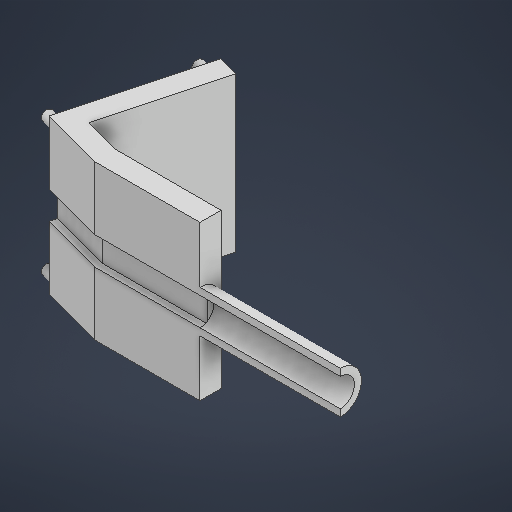
# Autodesk Inventor part: GY_906 Casetop
Saved by Autodesk Inventor 2027.1 (Build 311270010, 270A)
## iProperties
Created: 2026-09-10
Part Number: GY_906 Casetop
Material: Genérico
Document SubType Name: Modeling
Designer: marco
Density: 1 g/cm^3
Appearance: Valor por defecto
Author: marco
Autodesk Inventor part; units mm, degrees
ref_plane "YZ Plane" through (0, 0, 0) normal (1, 0, 0) x (0, 1, 0)
ref_plane "XZ Plane" through (0, 0, 0) normal (0, 1, 0) x (-1, 0, 0)
ref_plane "XY Plane" through (0, 0, 0) normal (0, 0, 1) x (1, 0, 0)
sketch "Boceto1" plane through (0, 0, 0) normal (0, 1, 0) x (-1, 0, 0)
  line L0 (0, 0) -> (-15, 0)
  line L1 (0, 0) -> (7.0223, -1.8816)
  line L2 (0, 0) -> (7.27, 0) construction
  line L3 (8.8653, -2.3754) -> (7.0223, -1.8816)
  line L4 (8.8653, -2.3754) -> (3.6889, -21.694)
  line L5 (8.8653, -2.3754) -> (28.8653, -2.3754) construction
  line L6 (-15, 0) -> (-15, -3)
  line L7 (-15, -3) -> (0, -3)
  line L8 (0, -3) -> (5.2175, -4.398)
  line L9 (5.2175, -4.398) -> (25.2175, -4.398) construction
  line L10 (3.6889, -21.694) -> (0.7911, -20.9175)
  line L11 (0.7911, -20.9175) -> (5.2175, -4.398)
  point P0 (4.2275, -19.6837)
  dimension "d0" = 15
  dimension "d1" = 7.27
  dimension "d2" = 15
  dimension "d3" = 1.908
  dimension "d4" = 20
  dimension "d5" = 105
  dimension "d7" = 3
  constraints: 24 end point, 4 horizontal, 2 equal length, 2 perpendicular, 1 collinear, 1 point on line, 1 vertical
  measures "d0" distance of L0.start L0.end
  measures "d1" distance of L0.start L1.end
  measures "d2" angle of L1 L2
  measures "d3" distance of L1.end L3.start
  measures "d4" distance of L3.start L4.end
  measures "d5" angle of L4 L5
  measures "d7" distance of L0.end L6.end
extrude "Extrusión1" add sketch "Boceto1" along normal blind 22
sketch "Boceto2" plane through (0, 0, 0) normal (-0.258819, 0, 0.9659258) x (0.9659258, 0, 0.258819)
  line L0 (-9.178, 0) -> (-9.178, 22) projected
  line L1 (-9.178, 0) -> (-9.178, 9)
  line L2 (-9.178, 9) -> (0, 9)
  line L3 (0, 9) -> (0, 13)
  line L4 (0, 13) -> (-9.178, 13)
  line L5 (-9.178, 13) -> (-9.178, 9)
  line L6 (0, 0) -> (0, 11)
  line L7 (0, 0) -> (0, 22) projected
  point P0 (-9.178, 13)
  dimension "d12" = 9
  dimension "d13" = 4
  dimension "d53" = 11
  constraints: 12 end point, 4 perpendicular, 2 point on line, 1 midpoint
  measures "d12" distance of L0.start L1.end
  measures "d13" distance of L2.end L3.end
  measures "d53" distance of L6.start L6.end
extrude "Extrusión2" cut sketch "Boceto2" against normal blind 1
sketch "Boceto3" plane through (0, 0, 0) normal (0, 0, 1) x (1, 0, 0)
  line L0 (15, 0) -> (15, 22) projected
  line L1 (15, 7) -> (15, 3.2945)
  line L2 (15, 3.2945) -> (15, 3)
  line L3 (15, 22) -> (0, 22) projected
  line L4 (15, 22) -> (15, 11)
  line L5 (15, 0) -> (15, 22) projected
  line L6 (0, 0) -> (0, 22) projected
  line L7 (13.0524, 11) -> (13.0524, 9)
  line L8 (13.0524, 9) -> (15, 9)
  line L9 (0, 9) -> (15, 9)
  line L10 (15, 11) -> (15, 13)
  line L11 (15, 13) -> (0, 13)
  point P0 (0, 9)
  point P1 (0, 13)
  dimension "d48" = 11
  dimension "d49" = 2
  dimension "d50" = 2
  constraints: 16 end point, 6 point on line, 3 perpendicular, 1 midpoint, 1 vertical
  measures "d48" distance of L0.end L4.end
  measures "d49" distance of L7.start L7.end
  measures "d50" distance of L4.end L10.end
sketch "Boceto7" plane through (-3.6889, 0, -21.694) normal (-0.9659258, 0, -0.258819) x (-0.258819, 0, 0.9659258)
  line L0 (0, 0) -> (0, 22) projected
  line L1 (0, 0) -> (0, 3)
  line L2 (0, 3) -> (20, 3)
  line L3 (20, 3) -> (20, 19)
  line L4 (20, 13) -> (20, 22) projected
  line L5 (20, 19) -> (17, 19)
  line L6 (17, 19) -> (17.1022, 3)
  line L7 (17.1022, 0) -> (17.1022, 22) projected
  line L8 (17, 19) -> (0, 19)
  line L9 (0, 22) -> (3, 22)
  line L10 (17.1022, 22) -> (0, 22) projected
  line L11 (3, 22) -> (3, 0)
  point P0 (20, 0)
  point P1 (20, 7)
  point P2 (3, 19)
  point P3 (3, 3)
  dimension "d30" = 3
  dimension "d31" = 16
  dimension "d32" = 3
  dimension "d33" = 3
  constraints: 16 end point, 8 point on line, 3 perpendicular
  measures "d30" distance of L0.start L1.end
  measures "d31" distance of L2.end L3.end
  measures "d32" distance of L3.end L5.end
  measures "d33" distance of L9.start L9.end
extrude "Extrusión6" add sketch "Boceto7" along normal blind 2 contours L11 L8 L6 L2
fillet "Empalme1" radius 1 4 edges at (-6.3972, 11, -19.3138) (-8.2222, 3, -12.503) (-10.0339, 11, -5.7415) (-8.2089, 19, -12.5523)
sketch "Boceto8" plane through (-3.6889, 0, -21.694) normal (-0.9659258, 0, -0.258819) x (-0.258819, 0, 0.9659258)
  line L0 (0, 0) -> (20, 0) projected
  line L1 (0, 0) -> (0, 1.5)
  line L2 (0, 0) -> (0, 22) projected
  line L3 (0, 1.5) -> (1.5, 1.5)
  line L4 (1.5, 1.5) -> (1.5, 20.5)
  line L5 (1.5, 20.5) -> (19, 20.5)
  line L6 (20, 13) -> (20, 22) projected
  line L7 (19, 20.5) -> (19, 1.5)
  line L8 (19, 1.5) -> (1.5, 1.5)
  circle A0 centre (1.5, 1.5) radius 0.75
  circle A1 centre (1.5, 20.5) radius 0.75
  circle A2 centre (19, 20.5) radius 0.75
  circle A3 centre (19, 1.5) radius 0.75
  dimension "d37" = 1.5
  dimension "d38" = 1.5
  dimension "d39" = 19
  dimension "d40" = 17.5
  dimension "d41" = 19
  dimension "d42" = 1.5
  dimension "d43" = 1.5
  dimension "d44" = 1.5
  dimension "d45" = 1.5
  constraints: 12 end point, 4 centre point, 4 coincident, 4 perpendicular, 2 point on line
  measures "d37" distance of L0.start L1.end
  measures "d38" distance of L1.end L3.end
  measures "d39" distance of L3.end L4.end
  measures "d40" distance of L4.end L5.end
  measures "d41" distance of L5.end L7.end
  measures "d42" diameter of A0
  measures "d43" diameter of A1
  measures "d44" diameter of A2
  measures "d45" diameter of A3
extrude "Extrusión7" add sketch "Boceto8" along normal blind 2 contours A0 L4 L3 | L3 L8 A0 | L4 A0 L8 | A1 L5 L4 | L4 L5 A1 | A3 L7 L8 | L8 L7 A3 | A2 L7 L5 | L5 L7 A2
extrude "Extrusión8" cut sketch "Boceto3" against normal blind 1 contours L8 L9 L6 L11 L0
sketch "Boceto9" plane through (15, 0, 0) normal (1, 0, 0) x (0, 0, -1)
  line L0 (0, 13) -> (0, 11)
  circle A0 centre (0, 11) radius 3
  circle A1 centre (0, 11) radius 2
  line L1 (0, 15.8082) -> (0, 4.1439)
  point P0 (0, 0)
  point P1 (0, 9)
  point P2 (0, 8)
  point P3 (0, 14)
  dimension "d54" = 2
  dimension "d55" = 4
  constraints: 4 end point, 2 centre point, 2 coincident, 2 vertical
  measures "d54" distance of L0.start L0.end
  measures "d55" diameter of A1
extrude "Extrusión9" add sketch "Boceto9" along normal blind 20 contours L1 A0 A1 picked at (2.6416, 11.2225)
